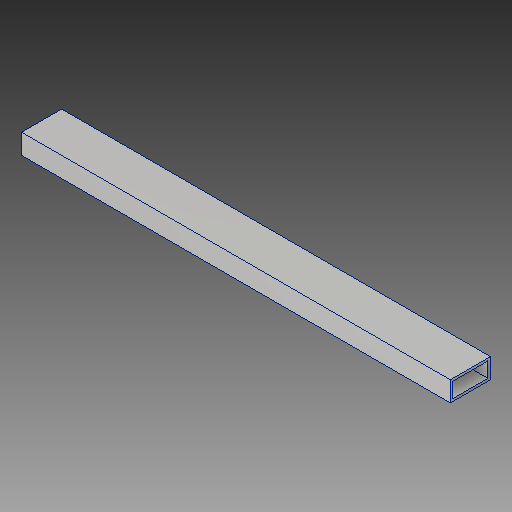
# Autodesk Inventor part: 1x2_alumTubing
Saved by Autodesk Inventor 2017 (Build 210142000, 142)
## iProperties
Created: 2016-02-15
Part Number: 1x2_alumTubing
Material: Aluminum 6061
Document SubType Name: Modeling
Designer: steele
Mass: 486.696 g
Surface Area: 1141.93 cm^2
Volume: 180.258 cm^3
Density: 2.7 g/cm^3
Appearance: Aluminum - Flat
Author: steele
Autodesk Inventor part; units mm, degrees
ref_plane "YZ Plane" through (0, 0, 0) normal (1, 0, 0) x (0, 1, 0)
ref_plane "XZ Plane" through (0, 0, 0) normal (0, 1, 0) x (-1, 0, 0)
ref_plane "XY Plane" through (0, 0, 0) normal (0, 0, 1) x (1, 0, 0)
sketch "Sketch1" plane through (0, 0, 0) normal (1, 0, 0) x (0, 1, 0)
  line L0 (-12.7, 25.4) -> (-12.7, -25.4)
  line L1 (-12.7, -25.4) -> (12.7, -25.4)
  line L2 (12.7, -25.4) -> (12.7, 25.4)
  line L3 (12.7, 25.4) -> (-12.7, 25.4)
  line L4 (-12.7, 25.4) -> (12.7, -25.4) construction
  line L5 (-12.7, -25.4) -> (12.7, 25.4) construction
  line L6 (-9.525, 22.225) -> (-9.525, -22.225)
  line L7 (-9.525, -22.225) -> (9.525, -22.225)
  line L8 (9.525, -22.225) -> (9.525, 22.225)
  line L9 (9.525, 22.225) -> (-9.525, 22.225)
  line L10 (-9.525, 22.225) -> (9.525, -22.225) construction
  line L11 (-9.525, -22.225) -> (9.525, 22.225) construction
  point P0 (0, 0)
  dimension "d0" = 25.4
  dimension "d1" = 50.8
  dimension "d2" = 3.175
  dimension "d3" = 3.175
  constraints: 24 end point, 4 midpoint, 4 parallel, 2 perpendicular, 2 vertical
  measures "d0" distance of L2.end L0.start
  measures "d1" distance of L0.start L0.end
  measures "d2" distance between parallel lines of L0 L6
  measures "d3" distance between parallel lines of L9 L3
extrude "Extrusion1" add sketch "Sketch1" along normal mid plane 542.925
equation "\"d0\" = width"
equation "\"d1\" = height"
equation "\"d2\" = wallThickness"
equation "\"d3\" = wallThickness"
equation "\"d4\" = length"
equation "\"width\" = 25.4"
equation "\"height\" = 50.8"
equation "\"length\" = 542.925"
equation "\"wallThickness\" = 3.175"
body "Solid1"
